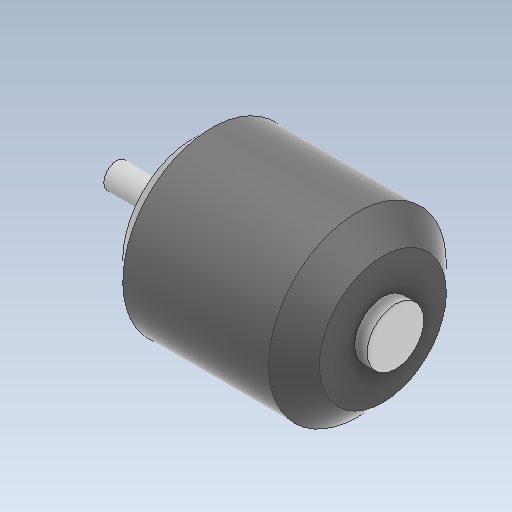
# Autodesk Inventor part: motor_sketch
Saved by Autodesk Inventor 2020 (Build 240168000, 168)
## iProperties
Created: 2024-02-19
Part Number: motor_sketch
Material: Типовые
Document SubType Name: Modeling
Designer: 4s
Density: 1 g/cm^3
Appearance: По умолчанию
Author: 4s
Autodesk Inventor part; units mm, degrees
ref_plane "YZ Plane" through (0, 0, 0) normal (1, 0, 0) x (0, 1, 0)
ref_plane "XZ Plane" through (0, 0, 0) normal (0, 1, 0) x (-1, 0, 0)
ref_plane "XY Plane" through (0, 0, 0) normal (0, 0, 1) x (1, 0, 0)
sketch "Эскиз1" plane through (0, 0, 0) normal (1, 0, 0) x (0, 1, 0)
  circle A0 centre (0, 0) radius 14
  dimension "d0" = 28
  constraints: 1 centre point, 1 coincident
  measures "d0" diameter of A0
extrude "Выдавливание1" add sketch "Эскиз1" along normal blind 18
sketch "Эскиз2" plane through (18, 0, 0) normal (1, 0, 0) x (0, 0, -1)
  circle A0 centre (0, 0) radius 14
  dimension "d3" = 28
  constraints: 1 centre point, 1 coincident
  measures "d3" diameter of A0
extrude "Выдавливание2" add sketch "Эскиз2" along normal blind 6
chamfer "Фаска1" distance 4 angle 45 1 edges at (24, 0, 14)
sketch "Эскиз3" plane through (24, 0, 0) normal (1, 0, 0) x (0, 0, -1)
  circle A0 centre (0, 0) radius 4.45
  dimension "d9" = 8.9
  constraints: 1 centre point, 1 coincident
  measures "d9" diameter of A0
extrude "Выдавливание3" add sketch "Эскиз3" along normal blind 2
sketch "Эскиз4" plane through (0, 0, 0) normal (-1, 0, 0) x (0, 0, 1)
  circle A0 centre (0, 0) radius 14
  dimension "d12" = 28
  constraints: 1 centre point, 1 coincident
  measures "d12" diameter of A0
extrude "Выдавливание4" add sketch "Эскиз4" along normal blind 6
chamfer "Фаска2" distance 3 angle 45 1 edges at (-6, 0, -14)
sketch "Эскиз5" plane through (-6, 0, 0) normal (-1, 0, 0) x (0, 0, 1)
  circle A0 centre (0, 0) radius 3.2
  dimension "d18" = 6.4
  constraints: 1 centre point, 1 coincident
  measures "d18" diameter of A0
extrude "Выдавливание5" add sketch "Эскиз5" along normal blind 1
sketch "Эскиз6" plane through (-7, 0, 0) normal (-1, 0, 0) x (0, 0, 1)
  circle A0 centre (0, 0) radius 2
  dimension "d21" = 4
  constraints: 1 centre point, 1 coincident
  measures "d21" diameter of A0
extrude "Выдавливание6" add sketch "Эскиз6" along normal blind 11
sketch "Эскиз7" plane through (-6, 0, 0) normal (-1, 0, 0) x (0, 0, 1)
  circle A0 centre (5.6569, 5.6569) radius 1.5
  line L0 (0, 0) -> (14, 0) construction
  circle A1 centre (0, 0) radius 14 construction
  line L1 (0, 0) -> (0, 14) construction
  line L2 (-4.7873, -4.7873) -> (5.6569, 5.6569) construction
  circle A2 centre (0, 0) radius 2 construction
  line L3 (-6.364, 6.364) -> (6.364, -6.364) construction
  circle A3 centre (-6.364, 6.364) radius 1.5
  circle A4 centre (6.364, -6.364) radius 1.5
  circle A5 centre (-5.6569, -5.6569) radius 1.5
  circle A6 centre (0, 0) radius 14 construction
  dimension "d24" = 3
  dimension "d29" = 45
  dimension "d30" = 3
  dimension "d31" = 16
  dimension "d32" = 18
  constraints: 8 end point, 5 centre point, 3 symmetric about line, 2 point on circle, 1 coincident, 1 horizontal, 1 midpoint, 1 point on line, 1 vertical, 3 other
  measures "d24" diameter of A0
  measures "d29" angle of L0 L2
  measures "d30" diameter of A3
  measures "d31" distance of A5.centre L2.end
  measures "d32" distance of L3.end L3.start
extrude "Выдавливание7" cut sketch "Эскиз7" against normal blind 6
